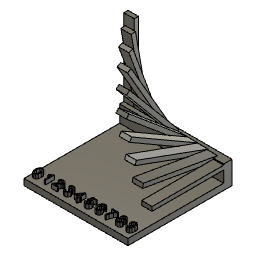
Overhang Test (Autodesk Fusion 360 design; units mm, degrees)
Autodesk Fusion 360 part; units mm, degrees
(part 1 of 6)
sketch "Sketch1" plane through (0, 0, 0) normal (0, 1, 0) x (1, 0, 0)
  line L0 (-25, 25) -> (25, 25)
  line L1 (25, 25) -> (25, -25)
  line L2 (25, -25) -> (-25, -25)
  line L3 (-25, -25) -> (-25, 25)
  constraint horizontal L0
  constraint vertical L1
  constraint horizontal L2
  constraint vertical L3
extrude "Extrude1" add sketch "Sketch1" along normal blind 3 makes body 1
sketch "Sketch2" plane through (0, 3, 0) normal (0, 1, 0) x (-1, 0, 0)
  line L0 (25, 25) -> (-25, 25)
  line L1 (-25, 25) -> (-25, -25)
  line L2 (-25, -25) -> (25, -25)
  line L3 (25, -25) -> (25, 25)
  line L4 (25, -25) -> (-25, -25)
  line L5 (-25, -25) -> (-25, -20)
  line L6 (-25, -20) -> (25, -20)
  line L7 (25, -20) -> (25, -25)
  constraint horizontal L4
  constraint vertical L5
  constraint horizontal L6
  constraint vertical L7
  constraint coincident L1 L5.end
  constraint coincident L2.end L3.start
extrude "Extrude2" add sketch "Sketch2" along normal blind 24 contours L1 L2 L3 L4 L5 L6 L7 bodies 1
sketch "Sketch3" plane through (0, 0, -20) normal (0, 0, 1) x (1, 0, 0)
  line L0 (-25, 3) -> (25, 3)
  line L1 (25, 3) -> (25, 27)
  line L2 (25, 27) -> (-25, 27)
  line L3 (-25, 27) -> (-25, 3)
  line L4 (-2, 25) -> (2, 25)
  line L5 (2, 25) -> (2, 20)
  line L6 (2, 20) -> (-2, 20)
  line L7 (-2, 20) -> (-2, 25)
  line L8 (5, 25) -> (9, 25)
  line L9 (9, 25) -> (9, 20)
  line L10 (9, 20) -> (5, 20)
  line L11 (5, 20) -> (5, 25)
  line L12 (12, 25) -> (16, 25)
  line L13 (16, 25) -> (16, 20)
  line L14 (16, 20) -> (12, 20)
  line L15 (12, 20) -> (12, 25)
  line L16 (19, 25) -> (23, 25)
  line L17 (23, 25) -> (23, 20)
  line L18 (23, 20) -> (19, 20)
  line L19 (19, 20) -> (19, 25)
  line L20 (-5, 25) -> (-9, 25)
  line L21 (-5, 20) -> (-5, 25)
  line L22 (-9, 20) -> (-5, 20)
  line L23 (-9, 25) -> (-9, 20)
  line L24 (-12, 20) -> (-12, 25)
  line L25 (-12, 25) -> (-16, 25)
  line L26 (-16, 25) -> (-16, 20)
  line L27 (-16, 20) -> (-12, 20)
  line L28 (-19, 20) -> (-19, 25)
  line L29 (-19, 25) -> (-23, 25)
  line L30 (-23, 25) -> (-23, 20)
  line L31 (-23, 20) -> (-19, 20)
  constraint horizontal L4
  constraint vertical L5
  constraint horizontal L6
  constraint vertical L7
  constraint horizontal L8
  constraint vertical L9
  constraint horizontal L10
  constraint vertical L11
  constraint horizontal L12
  constraint vertical L13
  constraint horizontal L14
  constraint vertical L15
  constraint horizontal L16
  constraint vertical L17
  constraint horizontal L18
  constraint vertical L19
sketch "Sketch4" plane through (0, 3, 0) normal (0, 1, 0) x (-1, 0, 0)
  line L0 (-25, -20) -> (25, -20)
  line L1 (25, -20) -> (25, 25)
  line L2 (25, 25) -> (-25, 25)
  line L3 (-25, 25) -> (-25, -20)
  line L4 (-19, -15) -> (-23, -15)
  line L5 (-23, -15) -> (-23, -11)
  line L6 (-23, -11) -> (-19, -11)
  line L7 (-19, -11) -> (-19, -15)
  line L8 (-16, -10) -> (-12, -10)
  line L9 (-12, -10) -> (-12, -6)
  line L10 (-12, -6) -> (-16, -6)
  line L11 (-16, -6) -> (-16, -10)
  line L12 (-9, -5) -> (-5, -5)
  line L13 (-5, -5) -> (-5, -1)
  line L14 (-5, -1) -> (-9, -1)
  line L15 (-9, -1) -> (-9, -5)
  line L16 (-2, 0) -> (2, 0)
  line L17 (2, 0) -> (2, 4)
  line L18 (2, 4) -> (-2, 4)
  line L19 (-2, 4) -> (-2, 0)
  line L20 (5, 5) -> (9, 5)
  line L21 (9, 5) -> (9, 9)
  line L22 (9, 9) -> (5, 9)
  line L23 (5, 9) -> (5, 5)
  line L24 (12, 10) -> (16, 10)
  line L25 (16, 10) -> (16, 14)
  line L26 (16, 14) -> (12, 14)
  line L27 (12, 14) -> (12, 10)
  line L28 (19, 15) -> (23, 15)
  line L29 (23, 15) -> (23, 19)
  line L30 (23, 19) -> (19, 19)
  line L31 (19, 19) -> (19, 15)
  constraint horizontal L4
  constraint vertical L5
  constraint horizontal L6
  constraint vertical L7
  constraint horizontal L8
  constraint vertical L9
  constraint horizontal L10
  constraint vertical L11
  constraint horizontal L12
  constraint vertical L13
  constraint horizontal L14
  constraint vertical L15
  constraint horizontal L16
  constraint vertical L17
  constraint horizontal L18
  constraint vertical L19
  constraint horizontal L20
  constraint vertical L21
  constraint horizontal L22
  constraint vertical L23
  constraint horizontal L24
  constraint vertical L25
  constraint horizontal L26
  constraint vertical L27
  constraint horizontal L28
  constraint vertical L29
  constraint horizontal L30
  constraint vertical L31
extrude "Extrude3" add sketch "Sketch4" along normal blind 22 contours L4 L5 L6 L7 | L8 L9 L10 L11 | L12 L13 L14 L15 | L16 L17 L18 L19 | L20 L21 L22 L23 | L24 L25 L26 L27 | L28 L29 L30 L31 bodies 1
extrude "Extrude4" add sketch "Sketch3" along normal blind 7 contours L4 L5 L6 L7 | L8 L9 L10 L11 | L12 L13 L14 L15 | L16 L17 L18 L19 | L20 L21 L22 L23 | L24 L25 L26 L27 | L28 L29 L30 L31 bodies 1
sketch "Sketch5" plane through (0, 20, 0) normal (0, -1, 0) x (1, 0, 0)
  line L0 (-12, -20) -> (-12, -13)
  line L1 (-12, -13) -> (-16, -13)
  line L2 (-16, -13) -> (-16, -20)
  line L3 (-16, -20) -> (-12, -20)
sketch "Sketch6" plane through (0, 0, -13) normal (0, 0, 1) x (1, 0, 0)
  line L0 (12, 20) -> (16, 20)
  line L1 (16, 20) -> (16, 25)
  line L2 (16, 25) -> (12, 25)
  line L3 (12, 25) -> (12, 20)
extrude "Extrude5" add sketch "Sketch6" along normal blind 5 bodies 1
sketch "Sketch7" plane through (0, 0, -13) normal (0, 0, 1) x (1, 0, 0)
  line L0 (5, 20) -> (9, 20)
  line L1 (9, 20) -> (9, 25)
  line L2 (9, 25) -> (5, 25)
  line L3 (5, 25) -> (5, 20)
extrude "Extrude6" add sketch "Sketch7" along normal blind 10 bodies 1
sketch "Sketch8" plane through (0, 0, -13) normal (0, 0, 1) x (1, 0, 0)
  line L0 (-2, 20) -> (2, 20)
  line L1 (2, 20) -> (2, 25)
  line L2 (2, 25) -> (-2, 25)
  line L3 (-2, 25) -> (-2, 20)
extrude "Extrude7" add sketch "Sketch8" along normal blind 13 bodies 1
sketch "Sketch9" plane through (0, 0, -13) normal (0, 0, 1) x (1, 0, 0)
  line L0 (-9, 25) -> (-9, 20)
  line L1 (-9, 20) -> (-5, 20)
  line L2 (-5, 20) -> (-5, 25)
  line L3 (-5, 25) -> (-9, 25)
extrude "Extrude8" add sketch "Sketch9" along normal blind 19 bodies 1
sketch "Sketch10" plane through (0, 0, -13) normal (0, 0, 1) x (1, 0, 0)
  line L0 (-16, 20) -> (-12, 20)
  line L1 (-12, 20) -> (-12, 25)
  line L2 (-12, 25) -> (-16, 25)
  line L3 (-16, 25) -> (-16, 20)
extrude "Extrude9" add sketch "Sketch10" along normal blind 25 bodies 1
sketch "Sketch11" plane through (0, 0, -13) normal (0, 0, 1) x (1, 0, 0)
  line L0 (-23, 20) -> (-19, 20)
  line L1 (-19, 20) -> (-19, 25)
  line L2 (-19, 25) -> (-23, 25)
  line L3 (-23, 25) -> (-23, 20)
extrude "Extrude10" add sketch "Sketch11" along normal blind 29 bodies 1
sketch "Sketch12" plane through (0, 3, 0) normal (0, 1, 0) x (-1, 0, 0)
  line L0 (-19, -11) -> (-19, -15)
  line L1 (-19, -15) -> (-23, -15)
  line L2 (-23, -15) -> (-23, -11)
  line L3 (-23, -11) -> (-19, -11)
  line L4 (5, 9) -> (9, 9)
  line L5 (9, 9) -> (9, 5)
  line L6 (9, 5) -> (5, 5)
  line L7 (5, 5) -> (5, 9)
  line L8 (12, 14) -> (16, 14)
  line L9 (16, 14) -> (16, 10)
  line L10 (16, 10) -> (12, 10)
  line L11 (12, 10) -> (12, 14)
  line L12 (-16, -6) -> (-12, -6)
  line L13 (-12, -6) -> (-12, -10)
  line L14 (-12, -10) -> (-16, -10)
  line L15 (-16, -10) -> (-16, -6)
  line L16 (-2, 4) -> (2, 4)
  line L17 (2, 4) -> (2, 0)
  line L18 (2, 0) -> (-2, 0)
  line L19 (-2, 0) -> (-2, 4)
  line L20 (19, 19) -> (23, 19)
  line L21 (23, 19) -> (23, 15)
  line L22 (23, 15) -> (19, 15)
  line L23 (19, 15) -> (19, 19)
  line L24 (-9, -1) -> (-5, -1)
  line L25 (-5, -1) -> (-5, -5)
  line L26 (-5, -5) -> (-9, -5)
  line L27 (-9, -5) -> (-9, -1)
  line L28 (-25, -20) -> (25, -20)
  line L29 (25, -20) -> (25, 25)
  line L30 (25, 25) -> (-25, 25)
  line L31 (-25, 25) -> (-25, -20)
  line L32 (23.4772, 23.7592) -> (-23.449, 23.7592) construction
  line L33 (-23.449, 23.7592) -> (-23.449, 18.7592) construction
  line L34 (-23.449, 18.7592) -> (23.4772, 18.7592) construction
  line L35 (23.4772, 18.7592) -> (23.4772, 23.7592) construction
  text T0 "35 30 25 20 15 10 05" font "Arial" height 5 bold align ink ink in box 0 x 0 at (23.4772, 23.7592) x (-1, 0) y (0, -1) spacing 1 height is em
  constraint perpendicular L32 L33
  constraint parallel L32 L34
  constraint parallel L33 L35
extrude "Extrude11" add sketch "Sketch12" along normal blind 2 text T0 bodies 1
sketch "Sketch13" plane through (0, 0, 0) normal (0, 1, 0) x (1, 0, 0)
  line L0 (50, 25) -> (100, 25)
  line L1 (100, 25) -> (100, -25)
  line L2 (100, -25) -> (50, -25)
  line L3 (50, -25) -> (50, 25)
  constraint horizontal L0
  constraint vertical L1
  constraint horizontal L2
  constraint vertical L3
extrude "Extrude12" add sketch "Sketch13" along normal blind 3 separate body makes body 2
sketch "Sketch14" plane through (0, 3, 0) normal (0, 1, 0) x (-1, 0, 0)
  line L0 (-50, 25) -> (-100, 25)
  line L1 (-100, 25) -> (-100, -25)
  line L2 (-100, -25) -> (-50, -25)
  line L3 (-50, -25) -> (-50, 25)
  line L4 (-50, -25) -> (-55, -25)
  line L5 (-55, -25) -> (-55, -20)
  line L6 (-55, -20) -> (-50, -20)
  line L7 (-50, -20) -> (-50, -25)
  constraint horizontal L4
  constraint vertical L5
  constraint horizontal L6
  constraint vertical L7
  constraint coincident L2.end L3.start
extrude "Extrude13" add sketch "Sketch14" along normal blind 37 separate body contours L2 L3 L4 L5 L6 L7 makes body 3
copy_body "CopyPasteBodies1" bodies 3 makes body 4
move_body "Move1" bodies 4 to x (1, 0, 0) y (0, 0.984808, 0.173648) z (0, -0.173648, 0.984808) at (5, -4.2956, -0.9008)
copy_body "CopyPasteBodies2" bodies 3 4 makes body 5 makes body 6
move_body "Move2" bodies 5 6 to x (1, 0, 0) y (0, 0.939693, 0.34202) z (0, -0.34202, 0.939693) at (10, -8.3696, -2.5337)
copy_body "CopyPasteBodies3" bodies 6 makes body 7
move_body "Move3" bodies 7 to x (1, 0, 0) y (0, 0.984808, 0.173648) z (0, -0.173648, 0.984808) at (5, -4.3336, -0.4666)
move_face "OffsetFaces1" offset -3 5 faces at (63.3333, 24.469, -11.865) (68.3333, 21.862, -8.3365) (73.3333, 18.6438, -4.8802) (58.3333, 26.4237, -15.7926) (53.3333, 27.6667, -20) on bodies 3 4 5 6 7
copy_body "CopyPasteBodies4" bodies 7 6 5 4 3 makes body 8 makes body 9 makes body 10 makes body 11 makes body 12
move_body "Move4" bodies 8 9 10 11 12 to x (1, 0, 0) y (0, 0.642788, 0.766044) z (0, -0.766044, 0.642788) at (25, -18.2197, -10.0595)
combine "Combine1" operation add target body 3 tool bodies 4 5 6 7 8 9 10 11 12
move_body "Move5" bodies 3 to x (1, 0, 0) y (0, 1, 0) z (0, 0, 1) at (0, 8, 0)
sketch "Sketch15" plane through (0, 3, 0) normal (0, 1, 0) x (-1, 0, 0)
  line L0 (-50, 25) -> (-100, 25)
  line L1 (-100, 25) -> (-100, -25)
  line L2 (-100, -25) -> (-50, -25)
  line L3 (-50, -25) -> (-50, 25)
  line L4 (-50, -25) -> (-100, -25)
  line L5 (-100, -25) -> (-100, -21)
  line L6 (-100, -21) -> (-50, -21)
  line L7 (-50, -21) -> (-50, -25)
  dimension "d28" = 4
  constraint horizontal L4
  constraint vertical L5
  constraint horizontal L6
  constraint vertical L7
  constraint coincident L2.end L3.start
  measures "d28" distance of L2.end L6.end
extrude "Extrude14" add sketch "Sketch15" along normal blind 8 contours L1 L2 L3 L4 L5 L6 L7 bodies 3 2
sketch "Sketch16" plane through (0, 3, 0) normal (0, 1, 0) x (-1, 0, 0)
  line L0 (-100, -21) -> (-50, -21)
  line L1 (-50, -21) -> (-50, 25)
  line L2 (-50, 25) -> (-100, 25)
  line L3 (-100, 25) -> (-100, -21)
  line L4 (-50.8818, 22.659) -> (-99.0078, 22.659) construction
  line L5 (-99.0078, 22.659) -> (-99.0078, 16.659) construction
  line L6 (-99.0078, 16.659) -> (-50.8818, 16.659) construction
  line L7 (-50.8818, 16.659) -> (-50.8818, 22.659) construction
  text T0 "0 1 2 3 4 5 6 7 8 9 " font "Arial" height 6 align ink ink in box 0 x 0 at (-50.8818, 22.659) x (-1, 0) y (0, -1) spacing 1 height is em
  constraint perpendicular L4 L5
  constraint parallel L4 L6
  constraint parallel L5 L7
extrude "Extrude15" add sketch "Sketch16" along normal blind 2 text T0 bodies 3
copy_body "CopyPasteBodies5" bodies 1 makes body 13
move_body "Move6" bodies 13 to x (1, 0, 0) y (0, 1, 0) z (0, 0, 1) at (-75, 0, 0)
move_face "OffsetFaces2" offset -5 1 faces at (-95.3333, 8.6667, 15) on bodies 13
move_face "OffsetFaces3" offset -7 1 faces at (-88.3333, 8.6667, 10) on bodies 13
move_face "OffsetFaces4" offset -5 1 faces at (-81.3333, 8.6667, 5) on bodies 13
move_face "OffsetFaces5" offset -5 1 faces at (-74.3333, 8.6667, 0) on bodies 13
move_face "OffsetFaces6" offset -7 1 faces at (-54.6667, 8.6667, -15) on bodies 13
move_face "OffsetFaces7" offset -7 1 faces at (-60.3333, 8.6667, -10) on bodies 13
move_face "OffsetFaces8" offset -7 1 faces at (-67.3333, 8.6667, -5) on bodies 13
move_face "OffsetFaces9" offset -4 7 faces at (-96.6667, 21.6667, 19) (-89.6667, 21.6667, 14) (-82.6667, 21.6667, 9) (-75.6667, 21.6667, 4) (-68.6667, 21.6667, -1) (-61.6667, 21.6667, -6) (-53.3333, 21.6667, -11) on bodies 13
move_body "Move7" bodies 13 to x (1, 0, 0) y (0, 1, 0) z (0, 0, 1) at (20, 0, 0)
move_body "Move8" bodies 3 to x (1, 0, 0) y (0, 1, 0) z (0, 0, 1) at (-20, 0, 0)
sketch "Sketch17" plane through (0, 0, 0) normal (0, 1, 0) x (1, 0, 0)
  line L0 (30, -30) -> (80, -30)
  line L1 (80, -30) -> (80, -80)
  line L2 (80, -80) -> (30, -80)
  line L3 (30, -80) -> (30, -30)
  constraint horizontal L0
  constraint vertical L1
  constraint horizontal L2
  constraint vertical L3
extrude "Extrude16" add sketch "Sketch17" along normal blind 3 separate body makes body 14
sketch "Sketch18" plane through (0, 3, 0) normal (0, 1, 0) x (-1, 0, 0)
  line L0 (-30, 80) -> (-80, 80)
  line L1 (-80, 80) -> (-80, 30)
  line L2 (-80, 30) -> (-30, 30)
  line L3 (-30, 30) -> (-30, 80)
  line L4 (-30, 80) -> (-80, 80)
  line L5 (-80, 80) -> (-80, 55)
  line L6 (-80, 55) -> (-30, 55)
  line L7 (-30, 55) -> (-30, 80)
  line L8 (-31, 31) -> (-32, 31)
  line L9 (-32, 31) -> (-32, 53)
  line L10 (-32, 53) -> (-31, 53)
  line L11 (-31, 53) -> (-31, 31)
  line L12 (-33, 31) -> (-34, 31)
  line L13 (-34, 31) -> (-34, 53)
  line L14 (-34, 53) -> (-33, 53)
  line L15 (-33, 53) -> (-33, 31)
  line L16 (-36, 31) -> (-37, 31)
  line L17 (-37, 31) -> (-37, 53)
  line L18 (-37, 53) -> (-36, 53)
  line L19 (-36, 53) -> (-36, 31)
  line L20 (-40, 31) -> (-41, 31)
  line L21 (-41, 31) -> (-41, 53)
  line L22 (-41, 53) -> (-40, 53)
  line L23 (-40, 53) -> (-40, 31)
  line L24 (-45, 31) -> (-46, 31)
  line L25 (-46, 31) -> (-46, 53)
  line L26 (-46, 53) -> (-45, 53)
  line L27 (-45, 53) -> (-45, 31)
  line L28 (-51, 31) -> (-52, 31)
  line L29 (-52, 31) -> (-52, 53)
  line L30 (-52, 53) -> (-51, 53)
  line L31 (-51, 53) -> (-51, 31)
  line L32 (-58, 31) -> (-59, 31)
  line L33 (-59, 31) -> (-59, 53)
  line L34 (-59, 53) -> (-58, 53)
  line L35 (-58, 53) -> (-58, 31)
  line L36 (-66, 31) -> (-67, 31)
  line L37 (-67, 31) -> (-67, 53)
  line L38 (-67, 53) -> (-66, 53)
  line L39 (-66, 53) -> (-66, 31)
  line L40 (-75, 31) -> (-76, 31)
  line L41 (-76, 31) -> (-76, 53)
  line L42 (-76, 53) -> (-75, 53)
  line L43 (-75, 53) -> (-75, 31)
  line L44 (-32, 79) -> (-32, 57)
  line L45 (-31, 79) -> (-32, 79)
  line L46 (-31, 57) -> (-31, 79)
  line L47 (-33, 57) -> (-33, 79)
  line L48 (-33, 79) -> (-34, 79)
  line L49 (-34, 79) -> (-34, 57)
  line L50 (-36, 57) -> (-36, 79)
  line L51 (-36, 79) -> (-37, 79)
  line L52 (-37, 79) -> (-37, 57)
  line L53 (-40, 57) -> (-40, 79)
  line L54 (-40, 79) -> (-41, 79)
  line L55 (-41, 79) -> (-41, 57)
  line L56 (-45, 57) -> (-45, 79)
  line L57 (-45, 79) -> (-46, 79)
  line L58 (-46, 79) -> (-46, 57)
  line L59 (-51, 57) -> (-51, 79)
  line L60 (-51, 79) -> (-52, 79)
  line L61 (-52, 79) -> (-52, 57)
  line L62 (-58, 57) -> (-58, 79)
  line L63 (-58, 79) -> (-59, 79)
  line L64 (-59, 79) -> (-59, 57)
  line L65 (-66, 57) -> (-66, 79)
  line L66 (-66, 79) -> (-67, 79)
  line L67 (-67, 79) -> (-67, 57)
  line L68 (-75, 57) -> (-75, 79)
  line L69 (-75, 79) -> (-76, 79)
  line L70 (-76, 79) -> (-76, 57)
  line L71 (-76, 57) -> (-75, 57)
  line L72 (-67, 57) -> (-66, 57)
  line L73 (-59, 57) -> (-58, 57)
  line L74 (-52, 57) -> (-51, 57)
  line L75 (-46, 57) -> (-45, 57)
  line L76 (-32, 57) -> (-31, 57)
  line L77 (-34, 57) -> (-33, 57)
  line L78 (-37, 57) -> (-36, 57)
  line L79 (-41, 57) -> (-40, 57)
  dimension "d43" = 25
  constraint horizontal L4
  constraint vertical L5
  constraint horizontal L6
  constraint vertical L7
  constraint coincident L0.start L3.end
  constraint horizontal L8
  constraint vertical L9
  constraint horizontal L10
  constraint vertical L11
  constraint horizontal L12
  constraint vertical L13
  constraint horizontal L14
  constraint vertical L15
  constraint horizontal L16
  constraint vertical L17
  constraint horizontal L18
  constraint vertical L19
  constraint horizontal L20
  constraint vertical L21
  constraint horizontal L22
  constraint vertical L23
  constraint horizontal L24
  constraint vertical L25
  constraint horizontal L26
  constraint vertical L27
  constraint horizontal L28
  constraint vertical L29
  constraint horizontal L30
  constraint vertical L31
  constraint horizontal L32
  constraint vertical L33
  constraint horizontal L34
  constraint vertical L35
  constraint horizontal L36
  constraint vertical L37
  constraint horizontal L38
  constraint vertical L39
  constraint horizontal L40
  constraint vertical L41
  constraint horizontal L42
  constraint vertical L43
  constraint symmetric L6 L8.start L45.start
  constraint symmetric L6 L8.end L44.start
  constraint symmetric L6 L9.end L44.end
  constraint symmetric L6 L10.end L46.start
  constraint symmetric L6 L12.start L47.end
  constraint symmetric L6 L12.end L48.end
  constraint symmetric L6 L13.end L49.end
  constraint symmetric L6 L14.end L47.start
  constraint symmetric L6 L16.start L50.end
  constraint symmetric L6 L16.end L51.end
  constraint symmetric L6 L17.end L52.end
  constraint symmetric L6 L18.end L50.start
  constraint symmetric L6 L20.start L53.end
  constraint symmetric L6 L20.end L54.end
  constraint symmetric L6 L21.end L55.end
  constraint symmetric L6 L22.end L53.start
  constraint symmetric L6 L24.start L56.end
  constraint symmetric L6 L24.end L57.end
  constraint symmetric L6 L25.end L58.end
  constraint symmetric L6 L26.end L56.start
  constraint symmetric L6 L28.start L59.end
  constraint symmetric L6 L28.end L60.end
  constraint symmetric L6 L29.end L61.end
  constraint symmetric L6 L30.end L59.start
  constraint symmetric L6 L32.start L62.end
  constraint symmetric L6 L32.end L63.end
  constraint symmetric L6 L33.end L64.end
  constraint symmetric L6 L34.end L62.start
  constraint symmetric L6 L36.start L65.end
  constraint symmetric L6 L36.end L66.end
  constraint symmetric L6 L37.end L67.end
  constraint symmetric L6 L38.end L65.start
  constraint symmetric L6 L40.start L68.end
  constraint symmetric L6 L40.end L69.end
  constraint symmetric L6 L41.end L70.end
  constraint symmetric L6 L42.end L68.start
  measures "d43" distance of L0.start L6.end
extrude "Extrude17" add sketch "Sketch18" along normal blind 5 contours L0 L1 L3 L4 L5 L6 L7 | L8 L9 L10 L11 | L12 L13 L14 L15 | L16 L17 L18 L19 | L20 L21 L22 L23 | L24 L25 L26 L27 | L28 L29 L30 L31 | L32 L33 L34 L35 | L36 L37 L38 L39 | L40 L41 L42 L43 bodies 14
sketch "Sketch19" plane through (0, 0, 0) normal (0, 1, 0) x (1, 0, 0)
  line L0 (-80, -30) -> (25, -30)
  line L1 (25, -30) -> (25, -80)
  line L2 (25, -80) -> (-80, -80)
  line L3 (-80, -80) -> (-80, -30)
  constraint horizontal L0
  constraint vertical L1
  constraint horizontal L2
  constraint vertical L3
extrude "Extrude18" add sketch "Sketch19" along normal blind 3 separate body makes body 15
sketch "Sketch20" plane through (0, 3, 0) normal (0, 1, 0) x (-1, 0, 0)
  line L0 (80, 80) -> (-25, 80)
  line L1 (-25, 80) -> (-25, 30)
  line L2 (-25, 30) -> (80, 30)
  line L3 (80, 30) -> (80, 80)
  line L4 (77.2573, 78.5659) -> (-11.4829, 78.5659) construction
  line L5 (-11.4829, 78.5659) -> (-11.4829, 58.5659) construction
  line L6 (-11.4829, 58.5659) -> (77.2573, 58.5659) construction
  line L7 (77.2573, 58.5659) -> (77.2573, 78.5659) construction
  text T0 "Enterprise" font "Arial" height 20 align ink ink in box 0 x 0 at (77.2573, 78.5659) x (-1, 0) y (0, -1) spacing 1 height is em
  constraint perpendicular L4 L5
  constraint parallel L4 L6
  constraint parallel L5 L7
extrude "Extrude19" add sketch "Sketch20" along normal blind 2 text T0 bodies 15
sketch "Sketch21" plane through (0, 3, 0) normal (0, 1, 0) x (-1, 0, 0)
  line L0 (77.2473, 74.5713) -> (77.2473, 60.2549)
  line L1 (77.2473, 60.2549) -> (66.8957, 60.2549)
  line L2 (66.8957, 60.2549) -> (66.8957, 61.9443)
  line L3 (66.8957, 61.9443) -> (75.3528, 61.9443)
  line L4 (75.3528, 61.9443) -> (75.3528, 66.3291)
  line L5 (75.3528, 66.3291) -> (67.4328, 66.3291)
  line L6 (67.4328, 66.3291) -> (67.4328, 68.0088)
  line L7 (67.4328, 68.0088) -> (75.3528, 68.0088)
  line L8 (75.3528, 68.0088) -> (75.3528, 72.8818)
  line L9 (75.3528, 72.8818) -> (66.5637, 72.8818)
  line L10 (66.5637, 72.8818) -> (66.5637, 74.5713)
  line L11 (66.5637, 74.5713) -> (77.2473, 74.5713)
  line L12 (49.2102, 72.999) -> (48.9563, 74.5517)
  spline S0 degree 3 poles (48.9563, 74.5517) (49.1899, 74.5972) (49.6288, 74.6827) (50.0755, 74.6999) (50.2844, 74.708) knots 0 0 0 0 0.071282 0.133904 0.133904 0.133904 0.133904
  spline S1 degree 3 poles (50.2844, 74.708) (50.5719, 74.7024) (51.0867, 74.6925) (51.5599, 74.4932) (51.7688, 74.4052) knots 0 0 0 0 0.085297 0.152712 0.152712 0.152712 0.152712
  spline S2 degree 3 poles (51.7688, 74.4052) (51.9303, 74.2993) (52.2429, 74.0941) (52.4236, 73.7673) (52.511, 73.6093) knots 0 0 0 0 0.056968 0.110293 0.110293 0.110293 0.110293
  spline S3 degree 3 poles (52.511, 73.6093) (52.5727, 73.3552) (52.738, 72.6752) (52.7305, 71.9736) (52.7258, 71.5341) knots 0 0 0 0 0.078216 0.209307 0.209307 0.209307 0.209307
  line L13 (52.7258, 71.5341) -> (52.7258, 65.5674)
  line L14 (52.7258, 65.5674) -> (54.0149, 65.5674)
  line L15 (54.0149, 65.5674) -> (54.0149, 64.2002)
  line L16 (54.0149, 64.2002) -> (52.7258, 64.2002)
  line L17 (52.7258, 64.2002) -> (52.7258, 61.6318)
  line L18 (52.7258, 61.6318) -> (50.9778, 60.5771)
  line L19 (50.9778, 60.5771) -> (50.9778, 64.2002)
  line L20 (50.9778, 64.2002) -> (49.2102, 64.2002)
  line L21 (49.2102, 64.2002) -> (49.2102, 65.5674)
  line L22 (49.2102, 65.5674) -> (50.9778, 65.5674)
  line L23 (50.9778, 65.5674) -> (50.9778, 71.6318)
  spline S4 degree 3 poles (50.9778, 71.6318) (50.9804, 71.8389) (50.9844, 72.1653) (50.9116, 72.4826) (50.885, 72.5986) knots 0 0 0 0 0.061811 0.09741 0.09741 0.09741 0.09741
  spline S5 degree 3 poles (50.885, 72.5986) (50.8488, 72.6668) (50.7753, 72.805) (50.6472, 72.8949) (50.5823, 72.9404) knots 0 0 0 0 0.022826 0.046239 0.046239 0.046239 0.046239
  spline S6 degree 3 poles (50.5823, 72.9404) (50.4984, 72.9773) (50.3077, 73.0612) (50.0987, 73.0651) (49.9817, 73.0674) knots 0 0 0 0 0.027232 0.061923 0.061923 0.061923 0.061923
  spline S7 degree 3 poles (49.9817, 73.0674) (49.8684, 73.0633) (49.6101, 73.0542) (49.354, 73.0188) (49.2102, 72.999) knots 0 0 0 0 0.033979 0.077495 0.077495 0.077495 0.077495
  line L24 (36.3879, 74.5713) -> (36.3879, 64.2002)
  line L25 (36.3879, 64.2002) -> (34.8059, 64.2002)
  line L26 (34.8059, 64.2002) -> (34.8059, 65.7724)
  spline S8 degree 3 poles (34.8059, 65.7724) (34.6297, 65.453) (34.3299, 64.9096) (33.8751, 64.4902) (33.6877, 64.3174) knots 0 0 0 0 0.1085 0.184546 0.184546 0.184546 0.184546
  spline S9 degree 3 poles (33.6877, 64.3174) (33.5128, 64.2148) (33.164, 64.0103) (32.7608, 63.9806) (32.5598, 63.9658) knots 0 0 0 0 0.059943 0.119555 0.119555 0.119555 0.119555
  spline S10 degree 3 poles (32.5598, 63.9658) (32.2553, 63.9939) (31.6135, 64.053) (31.0495, 64.3671) (30.7532, 64.5322) knots 0 0 0 0 0.090712 0.191197 0.191197 0.191197 0.191197
  line L27 (30.7532, 64.5322) -> (31.3586, 66.1631)
  spline S11 degree 3 poles (31.3586, 66.1631) (31.5689, 66.052) (31.9735, 65.8384) (32.4289, 65.8004) (32.6477, 65.7822) knots 0 0 0 0 0.070499 0.135652 0.135652 0.135652 0.135652
  spline S12 degree 3 poles (32.6477, 65.7822) (32.8348, 65.7966) (33.2089, 65.8254) (33.5249, 66.0278) (33.6828, 66.1289) knots 0 0 0 0 0.05537 0.110689 0.110689 0.110689 0.110689
  spline S13 degree 3 poles (33.6828, 66.1289) (33.8258, 66.2586) (34.1208, 66.5264) (34.2635, 66.8988) (34.3371, 67.0908) knots 0 0 0 0 0.057074 0.117791 0.117791 0.117791 0.117791
  spline S14 degree 3 poles (34.3371, 67.0908) (34.4226, 67.4162) (34.599, 68.0883) (34.6195, 68.7831) (34.6301, 69.1416) knots 0 0 0 0 0.100574 0.207758 0.207758 0.207758 0.207758
  line L28 (34.6301, 69.1416) -> (34.6301, 74.5713)
  line L29 (34.6301, 74.5713) -> (36.3879, 74.5713)
  line L30 (-9.6179, 71.2314) -> (-11.4343, 71.456)
  spline S15 degree 3 poles (-11.4343, 71.456) (-11.2675, 71.9516) (-10.9445, 72.9106) (-10.2016, 73.5957) (-9.8425, 73.9267) knots 0 0 0 0 0.154068 0.298151 0.298151 0.298151 0.298151
  spline S16 degree 3 poles (-9.8425, 73.9267) (-9.4126, 74.1828) (-8.4999, 74.7266) (-7.4364, 74.7783) (-6.8738, 74.8056) knots 0 0 0 0 0.147834 0.313845 0.313845 0.313845 0.313845
  spline S17 degree 3 poles (-6.8738, 74.8056) (-6.1659, 74.7587) (-4.8123, 74.669) (-3.765, 73.8128) (-3.2654, 73.4043) knots 0 0 0 0 0.206966 0.395783 0.395783 0.395783 0.395783
  spline S18 degree 3 poles (-3.2654, 73.4043) (-2.8772, 72.8627) (-2.0385, 71.6927) (-1.9695, 70.249) (-1.9324, 69.4736) knots 0 0 0 0 0.195785 0.422974 0.422974 0.422974 0.422974
  spline S19 degree 3 poles (-1.9324, 69.4736) (-1.9689, 68.6725) (-2.0368, 67.1854) (-2.8876, 65.9712) (-3.28, 65.4111) knots 0 0 0 0 0.234851 0.435929 0.435929 0.435929 0.435929
  spline S20 degree 3 poles (-3.28, 65.4111) (-3.7708, 64.9896) (-4.776, 64.1262) (-6.099, 64.0201) (-6.7761, 63.9658) knots 0 0 0 0 0.188967 0.387114 0.387114 0.387114 0.387114
  spline S21 degree 3 poles (-6.7761, 63.9658) (-7.433, 64.0198) (-8.7203, 64.1256) (-9.6965, 64.9688) (-10.1746, 65.3818) knots 0 0 0 0 0.192252 0.37676 0.37676 0.37676 0.37676
  spline S22 degree 3 poles (-10.1746, 65.3818) (-10.5585, 65.931) (-11.3913, 67.1223) (-11.4573, 68.5803) (-11.4929, 69.3662) knots 0 0 0 0 0.197018 0.427415 0.427415 0.427415 0.427415
  spline S23 degree 3 poles (-11.4929, 69.3662) (-11.4923, 69.4313) (-11.4908, 69.5876) (-11.486, 69.7438) (-11.4832, 69.8349) knots 0 0 0 0 0.019533 0.046886 0.046886 0.046886 0.046886
  line L31 (-11.4832, 69.8349) -> (-3.7488, 69.8349)
  spline S24 degree 3 poles (-3.7488, 69.8349) (-3.7996, 70.3557) (-3.8933, 71.3165) (-4.4573, 72.0954) (-4.7156, 72.4521) knots 0 0 0 0 0.153651 0.283492 0.283492 0.283492 0.283492
  spline S25 degree 3 poles (-4.7156, 72.4521) (-5.0252, 72.717) (-5.6501, 73.2517) (-6.4699, 73.3239) (-6.8836, 73.3603) knots 0 0 0 0 0.119065 0.24035 0.24035 0.24035 0.24035
  spline S26 degree 3 poles (-6.8836, 73.3603) (-7.1898, 73.3422) (-7.7821, 73.3072) (-8.2891, 73.0006) (-8.534, 72.8525) knots 0 0 0 0 0.090495 0.175003 0.175003 0.175003 0.175003
  spline S27 degree 3 poles (-8.534, 72.8525) (-8.7547, 72.6441) (-9.2382, 72.1877) (-9.4842, 71.5681) (-9.6179, 71.2314) knots 0 0 0 0 0.090002 0.197114 0.197114 0.197114 0.197114
  line L32 (80, 80) -> (-25, 80)
  line L33 (-25, 80) -> (-25, 30)
  line L34 (-25, 30) -> (80, 30)
  line L35 (80, 30) -> (80, 80)
  line L36 (64.1711, 74.5713) -> (64.1711, 64.2002)
  line L37 (64.1711, 64.2002) -> (62.5891, 64.2002)
  line L38 (62.5891, 64.2002) -> (62.5891, 65.6748)
  spline S28 degree 3 poles (62.5891, 65.6748) (62.1608, 65.1763) (61.2915, 64.1647) (59.9625, 64.0328) (59.2883, 63.9658) knots 0 0 0 0 0.189553 0.384716 0.384716 0.384716 0.384716
  spline S29 degree 3 poles (59.2883, 63.9658) (58.9854, 63.9785) (58.3935, 64.0032) (57.8366, 64.2045) (57.5647, 64.3027) knots 0 0 0 0 0.090359 0.176544 0.176544 0.176544 0.176544
  spline S30 degree 3 poles (57.5647, 64.3027) (57.3239, 64.4173) (56.8712, 64.6327) (56.5421, 65.0099) (56.3879, 65.1865) knots 0 0 0 0 0.078991 0.148563 0.148563 0.148563 0.148563
  spline S31 degree 3 poles (56.3879, 65.1865) (56.2667, 65.3814) (56.0155, 65.785) (55.9005, 66.2466) (55.841, 66.4853) knots 0 0 0 0 0.068412 0.1417 0.1417 0.1417 0.1417
  spline S32 degree 3 poles (55.841, 66.4853) (55.8129, 66.7089) (55.7414, 67.276) (55.7426, 67.8478) (55.7434, 68.1943) knots 0 0 0 0 0.067537 0.171325 0.171325 0.171325 0.171325
  line L39 (55.7434, 68.1943) -> (55.7434, 74.5713)
  line L40 (55.7434, 74.5713) -> (57.5012, 74.5713)
  line L41 (57.5012, 74.5713) -> (57.5012, 68.2627)
  spline S33 degree 3 poles (57.5012, 68.2627) (57.5029, 67.9476) (57.5058, 67.4028) (57.6468, 66.8776) (57.7063, 66.6562) knots 0 0 0 0 0.094012 0.162533 0.162533 0.162533 0.162533
  spline S34 degree 3 poles (57.7063, 66.6562) (57.7895, 66.4868) (57.959, 66.1415) (58.2736, 65.9196) (58.4338, 65.8066) knots 0 0 0 0 0.055666 0.113464 0.113464 0.113464 0.113464
  spline S35 degree 3 poles (58.4338, 65.8066) (58.6195, 65.7141) (59.0052, 65.5219) (59.436, 65.5004) (59.6594, 65.4892) knots 0 0 0 0 0.061552 0.127824 0.127824 0.127824 0.127824
  spline S36 degree 3 poles (59.6594, 65.4892) (60.0196, 65.5177) (60.7327, 65.5742) (61.3114, 65.9942) (61.5979, 66.2021) knots 0 0 0 0 0.106122 0.210147 0.210147 0.210147 0.210147
  spline S37 degree 3 poles (61.5979, 66.2021) (61.8341, 66.5354) (62.4018, 67.3364) (62.4091, 68.3281) (62.4133, 68.9072) knots 0 0 0 0 0.120022 0.288496 0.288496 0.288496 0.288496
  line L42 (62.4133, 68.9072) -> (62.4133, 74.5713)
  line L43 (62.4133, 74.5713) -> (64.1711, 74.5713)
  line L44 (40.3918, 71.2314) -> (38.5754, 71.456)
  spline S38 degree 3 poles (38.5754, 71.456) (38.7423, 71.9516) (39.0652, 72.9106) (39.8082, 73.5957) (40.1672, 73.9267) knots 0 0 0 0 0.154068 0.298151 0.298151 0.298151 0.298151
  spline S39 degree 3 poles (40.1672, 73.9267) (40.5971, 74.1828) (41.5099, 74.7266) (42.5734, 74.7783) (43.136, 74.8056) knots 0 0 0 0 0.147834 0.313845 0.313845 0.313845 0.313845
  spline S40 degree 3 poles (43.136, 74.8056) (43.8438, 74.7587) (45.1975, 74.669) (46.2447, 73.8128) (46.7444, 73.4043) knots 0 0 0 0 0.206966 0.395783 0.395783 0.395783 0.395783
  spline S41 degree 3 poles (46.7444, 73.4043) (47.1326, 72.8627) (47.9713, 71.6927) (48.0403, 70.249) (48.0774, 69.4736) knots 0 0 0 0 0.195785 0.422974 0.422974 0.422974 0.422974
  spline S42 degree 3 poles (48.0774, 69.4736) (48.0408, 68.6725) (47.973, 67.1854) (47.1222, 65.9712) (46.7297, 65.4111) knots 0 0 0 0 0.234851 0.435929 0.435929 0.435929 0.435929
  spline S43 degree 3 poles (46.7297, 65.4111) (46.239, 64.9896) (45.2337, 64.1262) (43.9108, 64.0201) (43.2336, 63.9658) knots 0 0 0 0 0.188967 0.387114 0.387114 0.387114 0.387114
  spline S44 degree 3 poles (43.2336, 63.9658) (42.5767, 64.0198) (41.2894, 64.1256) (40.3132, 64.9688) (39.8352, 65.3818) knots 0 0 0 0 0.192252 0.37676 0.37676 0.37676 0.37676
  spline S45 degree 3 poles (39.8352, 65.3818) (39.4513, 65.931) (38.6184, 67.1223) (38.5524, 68.5803) (38.5168, 69.3662) knots 0 0 0 0 0.197018 0.427415 0.427415 0.427415 0.427415
  spline S46 degree 3 poles (38.5168, 69.3662) (38.5175, 69.4313) (38.5189, 69.5876) (38.5238, 69.7438) (38.5266, 69.8349) knots 0 0 0 0 0.019533 0.046886 0.046886 0.046886 0.046886
  line L45 (38.5266, 69.8349) -> (46.261, 69.8349)
  spline S47 degree 3 poles (46.261, 69.8349) (46.2102, 70.3557) (46.1165, 71.3165) (45.5525, 72.0954) (45.2942, 72.4521) knots 0 0 0 0 0.153651 0.283492 0.283492 0.283492 0.283492
  spline S48 degree 3 poles (45.2942, 72.4521) (44.9846, 72.717) (44.3597, 73.2517) (43.5399, 73.3239) (43.1262, 73.3603) knots 0 0 0 0 0.119065 0.24035 0.24035 0.24035 0.24035
  spline S49 degree 3 poles (43.1262, 73.3603) (42.8199, 73.3422) (42.2277, 73.3072) (41.7207, 73.0006) (41.4758, 72.8525) knots 0 0 0 0 0.090495 0.175003 0.175003 0.175003 0.175003
  spline S50 degree 3 poles (41.4758, 72.8525) (41.255, 72.6441) (40.7715, 72.1877) (40.5255, 71.5681) (40.3918, 71.2314) knots 0 0 0 0 0.090002 0.197114 0.197114 0.197114 0.197114
  line L46 (18.6047, 74.5713) -> (18.6047, 64.2002)
  line L47 (18.6047, 64.2002) -> (17.0227, 64.2002)
  line L48 (17.0227, 64.2002) -> (17.0227, 65.7724)
  spline S51 degree 3 poles (17.0227, 65.7724) (16.8465, 65.453) (16.5467, 64.9096) (16.0919, 64.4902) (15.9045, 64.3174) knots 0 0 0 0 0.1085 0.184546 0.184546 0.184546 0.184546
  spline S52 degree 3 poles (15.9045, 64.3174) (15.7296, 64.2148) (15.3808, 64.0103) (14.9776, 63.9806) (14.7766, 63.9658) knots 0 0 0 0 0.059943 0.119555 0.119555 0.119555 0.119555
  spline S53 degree 3 poles (14.7766, 63.9658) (14.4721, 63.9939) (13.8303, 64.053) (13.2663, 64.3671) (12.97, 64.5322) knots 0 0 0 0 0.090712 0.191197 0.191197 0.191197 0.191197
  line L49 (12.97, 64.5322) -> (13.5754, 66.1631)
  spline S54 degree 3 poles (13.5754, 66.1631) (13.7857, 66.052) (14.1903, 65.8384) (14.6457, 65.8004) (14.8645, 65.7822) knots 0 0 0 0 0.070499 0.135652 0.135652 0.135652 0.135652
  spline S55 degree 3 poles (14.8645, 65.7822) (15.0516, 65.7966) (15.4257, 65.8254) (15.7417, 66.0278) (15.8996, 66.1289) knots 0 0 0 0 0.05537 0.110689 0.110689 0.110689 0.110689
  spline S56 degree 3 poles (15.8996, 66.1289) (16.0426, 66.2586) (16.3376, 66.5264) (16.4803, 66.8988) (16.5539, 67.0908) knots 0 0 0 0 0.057074 0.117791 0.117791 0.117791 0.117791
  spline S57 degree 3 poles (16.5539, 67.0908) (16.6394, 67.4162) (16.8158, 68.0883) (16.8363, 68.7831) (16.8469, 69.1416) knots 0 0 0 0 0.100574 0.207758 0.207758 0.207758 0.207758
  line L50 (16.8469, 69.1416) -> (16.8469, 74.5713)
  line L51 (16.8469, 74.5713) -> (18.6047, 74.5713)
  line L52 (11.9153, 74.5713) -> (11.9153, 64.2002)
  line L53 (11.9153, 64.2002) -> (10.1575, 64.2002)
  line L54 (10.1575, 64.2002) -> (10.1575, 74.5713)
  line L55 (10.1575, 74.5713) -> (11.9153, 74.5713)
  line L56 (8.1848, 71.4756) -> (6.4465, 71.2021)
  spline S58 degree 3 poles (6.4465, 71.2021) (6.3824, 71.5245) (6.2606, 72.1366) (5.8334, 72.5894) (5.6311, 72.8037) knots 0 0 0 0 0.096356 0.182984 0.182984 0.182984 0.182984
  spline S59 degree 3 poles (5.6311, 72.8037) (5.3709, 72.9657) (4.8009, 73.3208) (4.1272, 73.3464) (3.761, 73.3603) knots 0 0 0 0 0.090416 0.19813 0.19813 0.19813 0.19813
  spline S60 degree 3 poles (3.761, 73.3603) (3.3996, 73.352) (2.7562, 73.3372) (2.2055, 73.0104) (1.9641, 72.8672) knots 0 0 0 0 0.106187 0.189111 0.189111 0.189111 0.189111
  spline S61 degree 3 poles (1.9641, 72.8672) (1.7933, 72.7006) (1.4651, 72.3805) (1.4063, 71.9272) (1.3782, 71.7099) knots 0 0 0 0 0.069303 0.133141 0.133141 0.133141 0.133141
  spline S62 degree 3 poles (1.3782, 71.7099) (1.4008, 71.5213) (1.4465, 71.1393) (1.7448, 70.8957) (1.8957, 70.7724) knots 0 0 0 0 0.054773 0.110892 0.110892 0.110892 0.110892
  spline S63 degree 3 poles (1.8957, 70.7724) (2.104, 70.6789) (2.6816, 70.4195) (3.2983, 70.2714) (3.6926, 70.1767) knots 0 0 0 0 0.068379 0.189643 0.189643 0.189643 0.189643
  spline S64 degree 3 poles (3.6926, 70.1767) (4.2428, 70.0389) (5.1537, 69.8107) (6.0273, 69.4678) (6.3733, 69.332) knots 0 0 0 0 0.169911 0.281309 0.281309 0.281309 0.281309
  spline S65 degree 3 poles (6.3733, 69.332) (6.6051, 69.2051) (7.0553, 68.9589) (7.3589, 68.5459) (7.5061, 68.3457) knots 0 0 0 0 0.078215 0.151833 0.151833 0.151833 0.151833
  spline S66 degree 3 poles (7.5061, 68.3457) (7.6186, 68.1292) (7.8455, 67.6927) (7.8763, 67.2016) (7.8918, 66.9541) knots 0 0 0 0 0.072323 0.145834 0.145834 0.145834 0.145834
  spline S67 degree 3 poles (7.8918, 66.9541) (7.8791, 66.7281) (7.8538, 66.28) (7.667, 65.8721) (7.5744, 65.6699) knots 0 0 0 0 0.067242 0.133324 0.133324 0.133324 0.133324
  spline S68 degree 3 poles (7.5744, 65.6699) (7.459, 65.4813) (7.2281, 65.1038) (6.8829, 64.8269) (6.7102, 64.6884) knots 0 0 0 0 0.065793 0.131657 0.131657 0.131657 0.131657
  spline S69 degree 3 poles (6.7102, 64.6884) (6.5517, 64.5887) (6.202, 64.3687) (5.8077, 64.244) (5.592, 64.1757) knots 0 0 0 0 0.055946 0.123455 0.123455 0.123455 0.123455
  spline S70 degree 3 poles (5.592, 64.1757) (5.3487, 64.1145) (4.8503, 63.9891) (4.3365, 63.9737) (4.0735, 63.9658) knots 0 0 0 0 0.075035 0.153702 0.153702 0.153702 0.153702
  spline S71 degree 3 poles (4.0735, 63.9658) (3.6883, 63.977) (2.9576, 63.9983) (2.2599, 64.2149) (1.9299, 64.3174) knots 0 0 0 0 0.11496 0.218119 0.218119 0.218119 0.218119
  spline S72 degree 3 poles (1.9299, 64.3174) (1.649, 64.4364) (1.1263, 64.6578) (0.7443, 65.076) (0.5676, 65.2695) knots 0 0 0 0 0.090247 0.167948 0.167948 0.167948 0.167948
  spline S73 degree 3 poles (0.5676, 65.2695) (0.4307, 65.4984) (0.1328, 65.9966) (0.022, 66.5674) (-0.0379, 66.8759) knots 0 0 0 0 0.079396 0.172838 0.172838 0.172838 0.172838
  line L57 (-0.0379, 66.8759) -> (1.6809, 67.1103)
  spline S74 degree 3 poles (1.6809, 67.1103) (1.7352, 66.8607) (1.8405, 66.3773) (2.1904, 66.0288) (2.3596, 65.8603) knots 0 0 0 0 0.074855 0.144953 0.144953 0.144953 0.144953
  spline S75 degree 3 poles (2.3596, 65.8603) (2.5799, 65.7296) (3.067, 65.4406) (3.6353, 65.4215) (3.9465, 65.4111) knots 0 0 0 0 0.075664 0.167297 0.167297 0.167297 0.167297
  spline S76 degree 3 poles (3.9465, 65.4111) (4.3003, 65.414) (4.9097, 65.4189) (5.4488, 65.6955) (5.675, 65.8115) knots 0 0 0 0 0.104241 0.179577 0.179577 0.179577 0.179577
  spline S77 degree 3 poles (5.675, 65.8115) (5.8258, 65.9449) (6.1111, 66.1972) (6.1665, 66.5723) (6.1926, 66.749) knots 0 0 0 0 0.05827 0.110201 0.110201 0.110201 0.110201
  spline S78 degree 3 poles (6.1926, 66.749) (6.1835, 66.8603) (6.1652, 67.0839) (6.0404, 67.2705) (5.9778, 67.3642) knots 0 0 0 0 0.032912 0.066134 0.066134 0.066134 0.066134
  spline S79 degree 3 poles (5.9778, 67.3642) (5.8903, 67.4568) (5.6987, 67.6593) (5.4429, 67.7719) (5.3039, 67.833) knots 0 0 0 0 0.037826 0.08282 0.08282 0.08282 0.08282
  spline S80 degree 3 poles (5.3039, 67.833) (5.1308, 67.8875) (4.6169, 68.0495) (4.0964, 68.1894) (3.7512, 68.2822) knots 0 0 0 0 0.054441 0.161656 0.161656 0.161656 0.161656
  spline S81 degree 3 poles (3.7512, 68.2822) (3.2203, 68.4232) (2.3405, 68.6568) (1.4871, 68.9725) (1.1487, 69.0976) knots 0 0 0 0 0.164675 0.27286 0.27286 0.27286 0.27286
  spline S82 degree 3 poles (1.1487, 69.0976) (0.9178, 69.213) (0.4663, 69.4388) (0.1473, 69.8295) (-0.0086, 70.0205) knots 0 0 0 0 0.076456 0.14952 0.14952 0.14952 0.14952
  spline S83 degree 3 poles (-0.0086, 70.0205) (-0.1309, 70.2417) (-0.3894, 70.7089) (-0.415, 71.2431) (-0.4285, 71.5244) knots 0 0 0 0 0.074822 0.158007 0.158007 0.158007 0.158007
  spline S84 degree 3 poles (-0.4285, 71.5244) (-0.4059, 71.815) (-0.3599, 72.4051) (-0.0653, 72.9189) (0.0842, 73.1797) knots 0 0 0 0 0.086284 0.175226 0.175226 0.175226 0.175226
  spline S85 degree 3 poles (0.0842, 73.1797) (0.2791, 73.426) (0.6826, 73.9358) (1.2635, 74.2292) (1.5637, 74.3808) knots 0 0 0 0 0.093067 0.192613 0.192613 0.192613 0.192613
  spline S86 degree 3 poles (1.5637, 74.3808) (1.9036, 74.5047) (2.6099, 74.762) (3.3614, 74.7907) (3.7512, 74.8056) knots 0 0 0 0 0.107841 0.22405 0.22405 0.22405 0.22405
  spline S87 degree 3 poles (3.7512, 74.8056) (4.3603, 74.7884) (5.46, 74.7574) (6.4089, 74.21) (6.8323, 73.9658) knots 0 0 0 0 0.179334 0.323794 0.323794 0.323794 0.323794
  spline S88 degree 3 poles (6.8323, 73.9658) (7.1559, 73.6374) (7.8437, 72.9395) (8.0667, 71.9824) (8.1848, 71.4756) knots 0 0 0 0 0.135648 0.28832 0.28832 0.28832 0.28832
  line L58 (11.9153, 62.2763) -> (11.9153, 60.2549)
  line L59 (11.9153, 60.2549) -> (10.1575, 60.2549)
  line L60 (10.1575, 60.2549) -> (10.1575, 62.2763)
  line L61 (10.1575, 62.2763) -> (11.9153, 62.2763)
  line L62 (29.7082, 78.5459) -> (29.7082, 64.2002)
  line L63 (29.7082, 64.2002) -> (28.1067, 64.2002)
  line L64 (28.1067, 64.2002) -> (28.1067, 65.5478)
  spline S89 degree 3 poles (28.1067, 65.5478) (27.9177, 65.304) (27.5563, 64.8377) (27.0628, 64.5152) (26.8274, 64.3613) knots 0 0 0 0 0.091799 0.17557 0.17557 0.17557 0.17557
  spline S90 degree 3 poles (26.8274, 64.3613) (26.5684, 64.246) (26.0189, 64.0015) (25.4171, 63.9781) (25.0989, 63.9658) knots 0 0 0 0 0.084252 0.178765 0.178765 0.178765 0.178765
  spline S91 degree 3 poles (25.0989, 63.9658) (24.673, 63.9917) (23.8395, 64.0425) (23.1113, 64.45) (22.7551, 64.6494) knots 0 0 0 0 0.126163 0.246958 0.246958 0.246958 0.246958
  spline S92 degree 3 poles (22.7551, 64.6494) (22.4352, 64.9057) (21.7786, 65.432) (21.4106, 66.1896) (21.2219, 66.5781) knots 0 0 0 0 0.121368 0.249146 0.249146 0.249146 0.249146
  spline S93 degree 3 poles (21.2219, 66.5781) (21.071, 67.0089) (20.7615, 67.8924) (20.7237, 68.8282) (20.7043, 69.3076) knots 0 0 0 0 0.136145 0.279187 0.279187 0.279187 0.279187
  spline S94 degree 3 poles (20.7043, 69.3076) (20.7248, 69.8173) (20.7643, 70.8033) (21.109, 71.7274) (21.2756, 72.1738) knots 0 0 0 0 0.151918 0.293913 0.293913 0.293913 0.293913
  spline S95 degree 3 poles (21.2756, 72.1738) (21.4833, 72.5711) (21.8896, 73.3481) (22.5923, 73.8712) (22.9358, 74.1269) knots 0 0 0 0 0.132578 0.259289 0.259289 0.259289 0.259289
  spline S96 degree 3 poles (22.9358, 74.1269) (23.2998, 74.3249) (24.0153, 74.7139) (24.827, 74.7754) (25.2258, 74.8056) knots 0 0 0 0 0.122747 0.241277 0.241277 0.241277 0.241277
  spline S97 degree 3 poles (25.2258, 74.8056) (25.5078, 74.792) (26.0568, 74.7653) (26.5588, 74.5428) (26.803, 74.4345) knots 0 0 0 0 0.083889 0.163269 0.163269 0.163269 0.163269
  spline S98 degree 3 poles (26.803, 74.4345) (27.0235, 74.305) (27.4546, 74.0517) (27.7877, 73.6791) (27.9504, 73.497) knots 0 0 0 0 0.076211 0.148977 0.148977 0.148977 0.148977
  line L65 (27.9504, 73.497) -> (27.9504, 78.5459)
  line L66 (27.9504, 78.5459) -> (29.7082, 78.5459)
  line L67 (75, 58.7016) -> (8.4448, 58.7016) construction
  line L68 (8.4448, 58.7016) -> (8.4448, 43.7016) construction
  line L69 (8.4448, 43.7016) -> (75, 43.7016) construction
  line L70 (75, 43.7016) -> (75, 58.7016) construction
  text T0 "Enterprise" font "Arial" height 15 align ink ink in box 0 x 0 at (75, 58.7016) x (-1, 0) y (0, -1) spacing 1 height is em
  constraint perpendicular L67 L68
  constraint parallel L67 L69
  constraint parallel L68 L70
extrude "Extrude20" add sketch "Sketch21" along normal blind 2 text T0 bodies 15